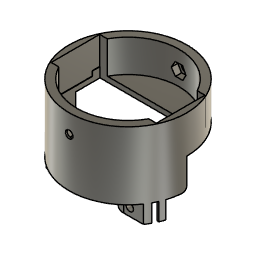
sensor_housing 3.0 v1 (Autodesk Fusion 360 design; units mm, degrees)
Autodesk Fusion 360 part; units mm, degrees
note: some values were not read from the file. Set by a fixed rule: which sketch regions a step uses.
sketch "sensor" plane through (0, 0, 3) normal (0, 0, 1) x (-1, 0, 0)
  circle A0 centre (0, 0) radius 30
  circle A1 centre (0, 0) radius 26.1 construction
  line L0 (-22.7, 10.31) -> (22.7, 10.31) construction
  line L1 (22.7, 10.31) -> (22.7, -10.31) construction
  line L2 (22.7, -10.31) -> (-22.7, -10.31) construction
  line L3 (-22.7, -10.31) -> (-22.7, 10.31) construction
  line L4 (-22.7, 10.31) -> (22.7, -10.31) construction
  line L5 (22.7, 10.31) -> (-22.7, -10.31) construction
  line L6 (-22.7, -10.31) -> (-21.1, -10.31) construction
  line L7 (-21.1, -10.31) -> (-21.1, -8.71) construction
  line L8 (-21.1, -8.71) -> (-22.7, -8.71) construction
  line L9 (-22.7, -8.71) -> (-22.7, -10.31) construction
  circle A2 centre (-21.1, -8.71) radius 0.75 construction
  line L10 (0, 0) -> (0, -6) construction
  line L11 (0, -6) -> (0, 0) construction
  line L12 (-6, 0) -> (0, 0) construction
  circle A3 centre (-21.1, 8.71) radius 0.75 construction
  circle A4 centre (21.1, -8.71) radius 0.75 construction
  circle A5 centre (21.1, 8.71) radius 0.75 construction
  circle A6 centre (0, 0) radius 26.1
  dimension "d4" = 52.2
  dimension "d5" = 45.4
  dimension "d6" = 20.62
  dimension "d76" = 1.6
  dimension "d77" = 1.6
  dimension "d78" = 1.5
  constraint concentric A0 A1
  constraint horizontal L0
  constraint perpendicular L0 L1
  constraint parallel L0 L2
  constraint parallel L1 L3
  constraint coincident L4 A0.centre
  constraint coincident L5 A0.centre
  constraint coincident A0.centre A1.centre
  constraint horizontal L6
  constraint vertical L7
  constraint horizontal L8
  constraint vertical L9
  constraint coincident L7.end L8.start
  constraint vertical L10
  constraint perpendicular L10 L12
  constraint symmetric A2 L12 A3
  constraint symmetric A2 L10 A4
  constraint symmetric L10 A3 A5
  measures "d4" diameter of A1
  measures "d5" distance of L1.end L2.end
  measures "d6" distance of L0.end L1.end
  measures "d76" distance of L2.end L6.end
  measures "d77" distance of L2.end L8.end
  measures "d78" diameter of A2
sketch "inner rim" plane through (0, 0, 0) normal (0, 0, -1) x (1, 0, 0)
  circle A0 centre (0, 0) radius 30
  circle A1 centre (0, 0) radius 25.75
  dimension "d7" = 51.5
  constraint concentric A0 A1
  measures "d7" diameter of A1
extrude "Extrude2" add sketch "inner rim" along normal blind 29.2 contours A1
sketch "sensor cavity" plane through (0, 0, 3) normal (0, 0, 1) x (1, 0, 0)
  line L0 (-22.75, 10.5) -> (-22.75, -10.5)
  line L1 (22.75, -10.5) -> (22.75, 10.5)
  line L2 (22.75, 10.5) -> (-22.75, -10.5) construction
  line L3 (-22.75, 10.5) -> (22.75, -10.5) construction
  line L4 (22.75, 10.5) -> (19.4358, 10.5)
  line L5 (-19.4358, 10.5) -> (-22.75, 10.5)
  line L6 (-22.75, -10.5) -> (-19.4358, -10.5)
  line L7 (19.4358, -10.5) -> (22.75, -10.5)
  arc A0 (19.4358, 10.5) -> (-19.4358, 10.5) centre (0, 0) ccw
  arc A1 (-19.4358, -10.5) -> (19.4358, -10.5) centre (0, 0) ccw
  dimension "d10" = 45.5
  dimension "d11" = 21
  constraint horizontal L4
  constraint perpendicular L0 L4
  constraint parallel L4 L6
  constraint parallel L0 L1
  constraint coincident L2 A0.centre
  constraint coincident L3 A0.centre
  constraint coincident A0.centre A1.centre
  constraint collinear L4 L5
  constraint coincident L6.end A0
  constraint coincident L7.start A0
  constraint collinear L6 L7
  constraint concentric A0 A1
  measures "d10" distance of L0.end L1.start
  measures "d11" distance of L0.start L0.end
extrude "Extrude3" cut sketch "sensor cavity" against normal blind 17
sketch "sensor hole" plane through (0, 0, -29.2) normal (0, 0, -1) x (1, 0, 0)
  circle A0 centre (0, 0) radius 25.75
  line L0 (0, 0) -> (0, 10.15) construction
  line L1 (0, 10.15) -> (0, 6.9) construction
  line L2 (0, 6.9) -> (8, 6.9)
  line L3 (8, 6.9) -> (8, 10.15)
  line L4 (8, 10.15) -> (-8, 10.15)
  line L5 (-8, 10.15) -> (-8, 6.9)
  line L6 (-8, 6.9) -> (0, 6.9)
  line L7 (0, 25) -> (0, 26.5) construction
  line L8 (0, 26.5) -> (0, 25.75) construction
  dimension "d14" = 10.15
  dimension "d49" = 3.25
  dimension "d50" = 8
  dimension "d51" = 3.25
  dimension "d52" = 16
  dimension "d53" = 3.25
  constraint coincident A0.centre L0.start
  constraint vertical L0
  constraint parallel L0 L1
  constraint perpendicular L0 L2
  constraint perpendicular L2 L3
  constraint perpendicular L3 L4
  constraint perpendicular L4 L5
  constraint vertical L7
  constraint midpoint L7 L8.end
  measures "d14" distance of A0.centre L0.end
  measures "d49" distance of L0.end L1.end
  measures "d50" distance of L1.end L2.end
  measures "d51" distance of L2.end L3.end
  measures "d52" distance of L3.end L4.end
  measures "d53" distance of L4.end L5.end
sketch "pcb" plane through (0, 0, -29.2) normal (0, 0, -1) x (1, 0, 0)
  circle A0 centre (0, 0) radius 25.75
  line L0 (0, 0) -> (0, 15.3788) construction
  line L1 (0, 15.3788) -> (0, 10.3) construction
  line L2 (0, 10.3) -> (0, 12.3) construction
  line L3 (-21.7798, 12.1192) -> (21.6502, 12.1192) construction
  line L4 (-21.7798, 12.1192) -> (-21.7798, 10.1192) construction
  line L5 (21.6502, 12.1192) -> (21.6502, 10.1192) construction
  line L6 (-0.0648, 12.1192) -> (-0.0648, 10.4192) construction
  line L7 (-6.4648, 10.4192) -> (-6.4648, 7.4192) construction
  line L8 (6.3352, 10.4192) -> (6.3352, 7.4192) construction
  line L9 (-6.4648, 7.4192) -> (6.3352, 7.4192) construction
  line L10 (-21.7798, 10.1192) -> (-6.4648, 10.1192) construction
  line L11 (6.3352, 10.1192) -> (21.6502, 10.1192) construction
  dimension "d39" = 2
  dimension "d40" = 43.43
  dimension "d41" = 2
  dimension "d42" = 43.43
  dimension "d43" = 1.7
  dimension "d44" = 6.4
  dimension "d45" = 6.4
  dimension "d46" = 3
  dimension "d47" = 3
  constraint coincident A0.centre L0.start
  constraint coincident L0 L1.end
  constraint parallel L1 L2
  constraint horizontal L3
  constraint perpendicular L3 L4
  constraint perpendicular L4 L10
  constraint midpoint L3 L6.start
  constraint perpendicular L3 L6
  constraint perpendicular L7 L10
  constraint perpendicular L8 L10
  constraint coincident L7 L10.end
  constraint coincident L8 L11.start
  constraint collinear L10 L11
  measures "d39" distance of L1.end L2.end
  measures "d40" distance of L3.start L3.end
  measures "d41" distance of L3.start L4.end
  measures "d42" distance of L4.end L5.end
  measures "d43" distance of L6.start L6.end
  measures "d44" distance of L6.end L8.start
  measures "d45" distance of L6.end L7.start
  measures "d46" distance of L7.start L7.end
  measures "d47" distance of L8.start L8.end
sketch "screw hole" plane through (0, 0, 0) normal (0, 1, 0) x (1, 0, 0)
  circle A0 centre (0, 8.1) radius 1.625
  line L0 (0, 0) -> (0, 8.1)
  dimension "d33" = 3.25
  dimension "d122" = 8.1
  constraint coincident L0.start origin
  constraint vertical L0
  constraint coincident A0.centre L0.end
  measures "d33" diameter of A0
  measures "d122" distance of L0.start A0.centre
extrude "Extrude6" cut sketch "screw hole" along normal mid plane 110
sketch "nut" plane through (0, 0, 0) normal (0, 1, 0) x (1, 0, 0)
  line L0 (1.5498, 5.3285) -> (3.1751, 8.0565)
  line L1 (3.1751, 8.0565) -> (1.6253, 10.828)
  line L2 (1.6253, 10.828) -> (-1.5498, 10.8715)
  line L3 (-1.5498, 10.8715) -> (-3.1751, 8.1435)
  line L4 (-3.1751, 8.1435) -> (-1.6253, 5.372)
  line L5 (-1.6253, 5.372) -> (1.5498, 5.3285)
  line L6 (0, 0) -> (0, 8.1) construction
  point P0 (0, 8.1)
  dimension "d36" = 2.75
  dimension "d123" = 8.1
  constraint coincident L6.start origin
  constraint vertical L6
  constraint coincident P0 L6.end
  measures "d36" distance of P0 L5
  measures "d123" distance of L6.start P0
extrude "Extrude7" cut sketch "nut" along normal mid plane 49.4
sketch "pcb holder" plane through (0, 0, -29.2) normal (0, 0, -1) x (1, 0, 0)
  arc A0 (22.5133, 12.4986) -> (21.3831, 14.3466) centre (0, 0) ccw
  circle A1 centre (0, 0) radius 25.75
  line L0 (-6.6, 9.9) -> (-6.6001, 9.9)
  line L1 (12.5003, 12.1) -> (22.73, 12.1)
  line L2 (12.5003, 14.35) -> (21.3831, 14.3466)
  arc A2 (22.73, 12.1) -> (21.3831, 14.3466) centre (0, 0) ccw
  line L3 (-12.5, 12.1) -> (-22.73, 12.1)
  line L4 (14.9761, 10.0342) -> (23.7145, 10.0342)
  line L5 (-10.3, 10.0342) -> (-23.6994, 10.0699)
  line L6 (-10.3, 7.85) -> (-24.5243, 7.85)
  arc A3 (-23.6994, 10.0699) -> (-24.5243, 7.85) centre (0, 0) ccw
  arc A4 (24.4786, 7.9912) -> (23.7145, 10.0342) centre (0, 0) ccw
  line L7 (-12.5, 14.35) -> (-21.3808, 14.35)
  arc A5 (-22.73, 12.1) -> (-21.3808, 14.35) centre (0, 0) ccw
  arc A6 (-21.3808, 14.35) -> (-22.73, 12.1) centre (0, 0) ccw
  line L8 (14.9761, 10.0342) -> (14.9761, 7.7842)
  line L9 (14.9761, 7.85) -> (24.5242, 7.8501)
  line L10 (-10.3, 10.0342) -> (-10.3, 7.85)
  line L11 (-12.5, 12.1) -> (12.5003, 12.1) construction
  line L12 (-10.3, 10.0342) -> (14.9761, 10.0342) construction
  line L13 (12.5003, 12.1) -> (10, 12.1)
  line L14 (10, 12.1) -> (10, 14.35)
  line L15 (10, 14.35) -> (12.5003, 14.35)
  line L16 (-12.5, 12.1) -> (-10.3, 12.1)
  line L17 (-12.5, 14.35) -> (-12.4999, 14.35)
  line L18 (-10.3, 12.1) -> (-10.3, 14.35)
  line L19 (-12.4999, 14.35) -> (-10.3, 14.35)
  dimension "d65" = 2.25
  dimension "d66" = 2.25
  dimension "d72" = 2.25
  dimension "d103" = 2.25
  dimension "d105" = 2.25
  constraint coincident A0.start A5
  constraint coincident L1.end A5
  constraint coincident A0.end A5
  constraint coincident L4.end A5
  constraint coincident A1 A4.start
  constraint coincident L5.end A5
  constraint horizontal L6
  constraint coincident L6.end A5
  constraint coincident A1 L7.end
  constraint perpendicular L4 L8
  constraint coincident L8 L9.start
  constraint coincident A1 L9.end
  constraint perpendicular L6 L10
  constraint perpendicular L8 L12
  constraint coincident A0.centre A1.centre
  constraint coincident L11 L13.end
  constraint perpendicular L13 L14
  constraint coincident L11 L16.end
  constraint perpendicular L11 L18
  constraint perpendicular L18 L19
  measures "d65" distance of L1.start L2.start
  measures "d66" distance of L3.start L7.start
  measures "d72" distance of L4.start L8.end
  measures "d103" distance of L13.end L14.end
  measures "d105" distance of L16.end L18.end
extrude "Extrude10" cut sketch "sensor hole" against normal blind 7 contours L2 L3 L4 L5 L6
sketch "wire cavity" plane through (0, 0, 3) normal (0, 0, 1) x (1, 0, 0)
  line L0 (0, -7) -> (0, -4) construction
  line L1 (-19.4358, -10.5) -> (-19.4358, -4)
  line L2 (-19.4358, -4) -> (0, -4)
  line L3 (19.4358, -10.5) -> (19.4358, -4)
  line L4 (19.4358, -4) -> (0, -4)
  arc A0 (-19.4358, -10.5) -> (19.4358, -10.5) centre (0, 0.1739) ccw
  point P0 (-22.75, -10.5)
  point P1 (-19.4358, -10.5)
  constraint vertical L0
  constraint vertical L1
  constraint symmetric L2.end L0 L4.end
  constraint symmetric L0 P1 L3.start
  constraint symmetric L0 L1.end L3.end
extrude "Extrude17" cut sketch "wire cavity" against normal blind 29
sketch "battery cavity" plane through (0, 0, -29.2) normal (0, 0, -1) x (1, 0, 0)
  line L0 (0, 0) -> (17.4, 0) construction
  line L1 (17.4, 0) -> (17.4, -17.2) construction
  line L2 (0, 0) -> (-17.4, 0) construction
  line L3 (-17.4, 0) -> (-17.4, -17.2) construction
  line L4 (-17.4, -17.2) -> (17.4, -17.2) construction
  line L5 (-25.75, 0) -> (25.75, 0)
  circle A0 centre (0, 0) radius 25.75
  arc A1 (-25.75, 0) -> (25.75, 0) centre (0, 0) ccw
  dimension "d94" = 17.4
  dimension "d95" = 17.2
  dimension "d96" = 17.4
  dimension "d97" = 17.2
  constraint coincident L0.start L2.start
  constraint horizontal L0
  constraint perpendicular L0 L1
  constraint parallel L0 L2
  constraint perpendicular L2 L3
  constraint perpendicular L1 L5
  constraint coincident L5.end A0
  constraint coincident L5.start A0
  measures "d94" distance of L0.start L0.end
  measures "d95" distance of L0.end L1.end
  measures "d96" distance of L0.start L2.end
  measures "d97" distance of L2.end L3.end
extrude "Extrude18" cut sketch "battery cavity" against normal blind 13 contours L5 A0 A1
sketch "sensor standoffs" plane through (0, 0, -14) normal (0, 0, 1) x (-1, 0, 0)
  line L0 (-19.4358, 4) -> (-19.4358, 10.5)
  line L1 (-19.4358, 10.5) -> (-22.75, 10.5)
  line L2 (-22.75, 10.5) -> (-22.75, -10.5)
  line L3 (22.75, -10.5) -> (22.75, 10.5)
  line L4 (22.75, 10.5) -> (19.4358, 10.5)
  line L5 (19.4358, 10.5) -> (19.4358, 4)
  line L6 (19.4358, 4) -> (0, 4)
  line L7 (0, 4) -> (-19.4358, 4)
  line L8 (22.75, 10.5) -> (19.4358, 10.5)
  line L9 (19.4358, 10.5) -> (19.4358, 7.25)
  line L10 (19.4358, 7.25) -> (22.75, 7.25)
  line L11 (22.75, 7.25) -> (22.75, 10.5)
  line L12 (0, 0) -> (0, -6)
  line L13 (-19.4358, 7.25) -> (-22.75, 7.25)
  line L14 (-19.4358, 10.5) -> (-19.4358, 7.25)
  line L15 (-22.75, 7.25) -> (-22.75, 10.5)
  line L16 (-22.75, 10.5) -> (-19.4358, 10.5)
  line L17 (-6, 0) -> (0, 0)
  line L18 (-22.75, -10.5) -> (-19.4358, -10.5)
  line L19 (-22.75, -7.25) -> (-22.75, -10.5)
  line L20 (-19.4358, -7.25) -> (-22.75, -7.25)
  line L21 (-19.4358, -10.5) -> (-19.4358, -7.25)
  line L22 (19.4358, -7.25) -> (22.75, -7.25)
  line L23 (19.4358, -10.5) -> (19.4358, -7.25)
  line L24 (22.75, -10.5) -> (19.4358, -10.5)
  line L25 (22.75, -7.25) -> (22.75, -10.5)
  line L26 (-22.75, -10.5) -> (-19.4358, -10.5)
  arc A0 (-19.4358, -10.5) -> (19.4358, -10.5) centre (0, 0) ccw
  line L27 (19.4358, -10.5) -> (22.75, -10.5)
  constraint horizontal L8
  constraint vertical L9
  constraint horizontal L10
  constraint vertical L11
  constraint midpoint L5 L9.end
  constraint coincident L3.end L4.start
  constraint symmetric L3.end L12 L1.end
  constraint symmetric L4.end L12 L0.end
  constraint symmetric L9.end L12 L13.start
  constraint symmetric L10.end L12 L13.end
  constraint symmetric L3.end L17 L3.start
  constraint symmetric L4.end L17 L23.start
  constraint symmetric L9.end L17 L22.start
  constraint symmetric L10.end L17 L22.end
  constraint symmetric L13.start L17 L20.start
  constraint symmetric L13.end L17 L19.start
  constraint symmetric L0.end L17 L18.end
  constraint symmetric L1.end L17 L2.end
extrude "Extrude19" add sketch "sensor standoffs" along normal blind 2 contours L0 L1 L2 L13 L14 L15 L16 | L2 L18 L19 L20 L21 L26 | L3 L4 L5 L8 L9 L10 L11 | L3 L22 L23 L24 L25 L27
sketch "hole offset" plane through (0, 0, -29.2) normal (0, 0, -1) x (1, 0, 0)
  line L0 (-25.75, 0) -> (25.75, 0)
  arc A0 (25.75, 0) -> (-25.75, 0) centre (0, 0) ccw
  line L1 (0, 10.15) -> (15.1099, 10.1) construction
  line L2 (15.1099, 14.349) -> (15.1099, 10.1) construction
  line L3 (8, 10.15) -> (8, 6.9)
  line L4 (8, 6.9) -> (-8, 6.9)
  line L5 (-8, 6.9) -> (-8, 10.15)
  line L6 (-8, 10.15) -> (8, 10.15)
  dimension "d102" = 15.11
  measures "d102" distance of L1.start L1.end
extrude "Extrude20" add sketch "pcb holder" along normal blind 7.62 contours A0 A1 L1 L2 A2 A5 L13 L14 L15 | A1 L3 L7 A6 L16 L18 L19 | A1 L4 A4 A5 L8 L9 | A1 L5 L6 A3 A5 L10
sketch "pcb mounting" plane through (0, -7.85, 0) normal (0.000006, 1, 0) x (-1, 0.000006, 0)
  line L0 (-14.9761, -29.2) -> (-24.5243, -29.2)
  line L1 (-24.5243, -29.2) -> (-24.5243, -36.82)
  line L2 (-24.5243, -36.82) -> (-14.9761, -36.82)
  line L3 (-14.9761, -36.82) -> (-14.9761, -29.2)
  line L4 (-15.11, -29.2) -> (-15.11, -33.4) construction
  circle A0 centre (-15.11, -33.4) radius 1.6
  line L5 (0, -43) -> (0, -49) construction
  circle A1 centre (15.11, -33.4) radius 1.6
  point P0 (-15.11, -29.2)
  dimension "d108" = 4.2
  dimension "d109" = 3.2
  constraint coincident L0 P0
  constraint perpendicular L0 L4
  constraint coincident P0 L4.start
  constraint coincident L4.end A0.centre
  constraint perpendicular L2 L5
  constraint symmetric A0 L5 A1
  measures "d108" distance of P0 L4.end
  measures "d109" diameter of A0
extrude "Extrude21" cut sketch "pcb mounting" against normal blind 9 contours L3 A0 | L3 A0 | A1
fillet "Fillet2" radius 2 1 edges at (0, 0, -29.2)
move_face "OffsetFaces1" offset 3 1 faces at (-21.3038, 12.0593, 0)
fillet "Fillet3" radius 2 3 edges at (-10.3, -8.9421, -36.82) (-10.3, -13.225, -36.82) (10, -13.225, -36.82)
sketch "Sketch21" plane through (0, 0, 3) normal (0, 0, 1) x (-1, 0, 0)
  line L0 (-22.75, 10.5) -> (-19.4358, 10.5)
  arc A0 (19.4358, 10.5) -> (-19.4358, 10.5) centre (0, 0) ccw
  line L1 (19.4358, 10.5) -> (22.75, 10.5)
  line L2 (22.75, 10.5) -> (22.75, -10.5)
  line L3 (22.75, -10.5) -> (19.4358, -10.5)
  arc A1 (-19.4358, -10.5) -> (19.4358, -10.5) centre (0, 0) ccw
  line L4 (-19.4358, -10.5) -> (-22.75, -10.5)
  line L5 (-22.75, -10.5) -> (-22.75, 10.5)
  circle A2 centre (0, 0) radius 25.75
  circle A3 centre (0, 0) radius 25.4402
  dimension "d126" = -0.3098
extrude "Extrude23" cut sketch "Sketch21" against normal blind 44 contours A2
sketch "Sketch22" plane through (0, 0, 0) normal (0, 0, 1) x (1, 0, 0)
  line L0 (22.605, 10.5) -> (-22.605, 10.5)
  line L1 (-22.605, 10.5) -> (-22.605, -10.5)
  line L2 (-22.605, -10.5) -> (22.605, -10.5)
  line L3 (22.605, -10.5) -> (22.605, 10.5)
  line L4 (22.605, 10.5) -> (-22.605, -10.5) construction
  line L5 (-22.605, 10.5) -> (22.605, -10.5) construction
  dimension "d129" = 45.21
  dimension "d130" = 21
  constraint horizontal L0
  constraint perpendicular L0 L1
  constraint parallel L0 L2
  constraint parallel L1 L3
  constraint coincident L4 origin
  constraint coincident L5 origin
  measures "d129" distance of L0.start L0.end
  measures "d130" distance of L0.end L1.end
extrude "Extrude24" cut sketch "Sketch22" along normal blind 0 and the other way through all
sketch "Sketch23" plane through (0, 0, 3) normal (0, 0, 1) x (-1, 0, 0)
  circle A0 centre (0, 0) radius 25.4402
  line L0 (-22.75, 10.5) -> (-19.4358, 10.5)
  arc A1 (19.4358, 10.5) -> (-19.4358, 10.5) centre (0, 0) ccw
  line L1 (19.4358, 10.5) -> (22.75, 10.5)
  line L2 (22.75, 10.5) -> (22.75, -10.5)
  line L3 (22.75, -10.5) -> (19.4358, -10.5)
  arc A2 (-19.4358, -10.5) -> (19.4358, -10.5) centre (0, 0) ccw
  line L4 (-19.4358, -10.5) -> (-22.75, -10.5)
  line L5 (-22.75, -10.5) -> (-22.75, 10.5)
  circle A3 centre (0, 0) radius 25.4402
  circle A4 centre (0, 0) radius 22.0907
  constraint coincident A0.centre A1.centre
  constraint concentric A3 A4
extrude "Extrude25" cut sketch "Sketch23" against normal blind 3
